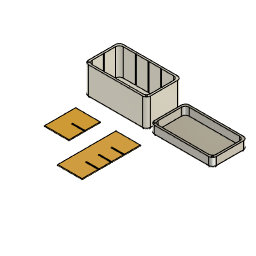
modularTreatBox v3 (Autodesk Fusion 360 design; units mm, degrees)
Autodesk Fusion 360 part; units mm, degrees
note: some values were not read from the file. Chosen so that the rebuilt part matches the saved one: which face or edge a step refers to.
sketch "Sketch1" plane through (0, 0, 0) normal (0, 0, 1) x (1, 0, 0)
  line L0 (65, 40) -> (-65, 40)
  line L1 (-75, 30) -> (-75, -30)
  line L2 (-65, -40) -> (65, -40)
  line L3 (75, -30) -> (75, 30)
  line L4 (-70, 45) -> (70, 45)
  line L5 (80, 35) -> (80, -35)
  line L6 (70, -45) -> (-70, -45)
  line L7 (-80, -35) -> (-80, 35)
  arc A0 (-65, 40) -> (-75, 30) centre (-65, 30) ccw
  arc A1 (-75, -30) -> (-65, -40) centre (-65, -30) ccw
  arc A2 (65, -40) -> (75, -30) centre (65, -30) ccw
  arc A3 (75, 30) -> (65, 40) centre (65, 30) ccw
  arc A4 (70, -45) -> (80, -35) centre (70, -35) ccw
  arc A5 (80, 35) -> (70, 45) centre (70, 35) ccw
  arc A6 (-70, 45) -> (-80, 35) centre (-70, 35) ccw
  arc A7 (-80, -35) -> (-70, -45) centre (-70, -35) ccw
  point P0 (75, 40)
  point P1 (-75, 40)
  point P2 (75, -40)
  point P3 (-80, 45)
  point P4 (80, 45)
  point P5 (-80, -45)
  dimension "d3" = 150
  dimension "d4" = 80
  dimension "d7" = 160
  dimension "d8" = 90
  dimension "d9" = 10
  dimension "d10" = 10
  dimension "d11" = 10
  constraint horizontal L0
  constraint vertical L1
  constraint horizontal L2
  constraint vertical L3
  constraint horizontal L4
  constraint vertical L5
  constraint horizontal L6
  constraint vertical L7
  constraint coincident P1 L0
  constraint coincident P1 L1
  constraint tangent L0 A0
  constraint tangent L1 A0
  constraint tangent L1 A1
  constraint tangent L2 A1
  constraint coincident P2 L2
  constraint coincident P2 L3
  constraint tangent L2 A2
  constraint tangent L3 A2
  constraint equal A1 A2
  constraint coincident P0 L0
  constraint coincident P0 L3
  constraint tangent L0 A3
  constraint tangent L3 A3
  constraint equal A1 A3
  constraint tangent L5 A4
  constraint tangent L6 A4
  constraint coincident P4 L4
  constraint coincident P4 L5
  constraint tangent L4 A5
  constraint tangent L5 A5
  constraint equal A4 A5
  constraint coincident P3 L4
  constraint coincident P3 L7
  constraint tangent L4 A6
  constraint tangent L7 A6
  constraint equal A4 A6
  constraint coincident P5 L6
  constraint coincident P5 L7
  constraint tangent L6 A7
  constraint tangent L7 A7
  constraint equal A4 A7
  measures "d3" distance of P0 P1
  measures "d4" distance of P0 P2
  measures "d7" distance of P3 P4
  measures "d8" distance of P3 P5
  measures "d9" radius of A0
  measures "d10" radius of A1
  measures "d11" radius of A4
extrude "Extrude1" add sketch "Sketch1" against normal blind 5 contours L0 L1 L2 L3 A0 A1 A2 A3 | L4 L5 L6 L7 A4 A5 A6 A7 makes body 1
extrude "Extrude2" add sketch "Sketch1" along normal blind 70 bodies 1
copy_body "CopyPasteBodies1" bodies 1 makes body 2
move_body "Move1" bodies 2 to x (1, 0, 0) y (0, 1, 0) z (0, 0, 1) at (170, 0, 0)
extrude "Extrude3" cut 1 faces at (191.6667, -43.3333, 70) along direction (0, 0, -1) blind 50 on bodies 2 bodies 2
sketch "Sketch2" plane through (0, 0, 70) normal (0, 0, 1) x (-1, 0, 0)
  arc A0 (-75, -30) -> (-65, -40) centre (-65, -30) ccw
  line L0 (-75, -30) -> (-75, 30)
  arc A1 (-65, 40) -> (-75, 30) centre (-65, 30) ccw
  line L1 (-65, 40) -> (65, 40)
  arc A2 (75, 30) -> (65, 40) centre (65, 30) ccw
  line L2 (75, 30) -> (75, -30)
  arc A3 (65, -40) -> (75, -30) centre (65, -30) ccw
  line L3 (65, -40) -> (-65, -40)
  arc A4 (70, -45) -> (80, -35) centre (70, -35) ccw
  line L4 (80, -35) -> (80, 35)
  arc A5 (80, 35) -> (70, 45) centre (70, 35) ccw
  line L5 (70, 45) -> (-70, 45)
  arc A6 (-70, 45) -> (-80, 35) centre (-70, 35) ccw
  line L6 (-80, 35) -> (-80, -35)
  arc A7 (-80, -35) -> (-70, -45) centre (-70, -35) ccw
  line L7 (-70, -45) -> (70, -45)
  line L8 (65, -40) -> (32.5, -40)
  line L9 (32.5, -40) -> (0, -40)
  line L10 (0, -40) -> (-32.5, -40)
  line L11 (-32.5, -40) -> (-65, -40)
  line L12 (32.5, -40) -> (32.5, 40)
  line L13 (0, -40) -> (0, 40)
  line L14 (-32.5, -40) -> (-32.5, 40)
  line L15 (-75, 0) -> (75, 0)
  arc A8 (75, -1.25) -> (75, 1.25) centre (75, 0) ccw
  arc A9 (31.25, -40) -> (33.75, -40) centre (32.5, -40) ccw
  arc A10 (-1.25, -40) -> (1.25, -40) centre (0, -40) ccw
  arc A11 (-33.75, -40) -> (-31.25, -40) centre (-32.5, -40) ccw
  arc A12 (-31.25, 40) -> (-33.75, 40) centre (-32.5, 40) ccw
  arc A13 (1.25, 40) -> (-1.25, 40) centre (0, 40) ccw
  arc A14 (33.75, 40) -> (31.25, 40) centre (32.5, 40) ccw
  arc A15 (-75, 1.25) -> (-75, -1.25) centre (-75, 0) ccw
  dimension "d18" = 32.5
  dimension "d19" = 32.5
  dimension "d20" = 32.5
  dimension "d21" = 1.25
  dimension "d22" = 1.25
  dimension "d23" = 1.25
  dimension "d24" = 1.25
  dimension "d25" = 1.25
  dimension "d26" = 1.25
  dimension "d27" = 1.25
  dimension "d28" = 1.25
  constraint coincident A3.start L3.start
  constraint parallel L3 L8
  constraint parallel L3 L9
  constraint parallel L3 L10
  constraint coincident A0.end L3.end
  constraint coincident L1 L12.end
  constraint perpendicular L1 L12
  constraint midpoint L1 L13.end
  constraint coincident L1 L14.end
  constraint perpendicular L1 L14
  constraint midpoint L0 L15.start
  constraint midpoint L2 L15.end
  constraint coincident L2 A8.end
  constraint coincident L2 A8.start
  constraint coincident L15.end A8.centre
  constraint coincident L8 A9.start
  constraint coincident L8.end L9.start
  constraint coincident L9 A10.start
  constraint coincident L9.end L10.start
  constraint coincident L10 A11.start
  constraint coincident L10.end L11.start
  constraint coincident L1 A12.start
  constraint coincident L14.end A12.centre
  constraint coincident L1 A13.start
  constraint coincident L13.end A13.centre
  constraint coincident L1 A14.start
  constraint coincident L12.end A14.centre
  constraint coincident L0 A15.start
  constraint coincident L15.start A15.centre
  measures "d18" distance of A3.start L8.end
  measures "d19" distance of L8.end L9.end
  measures "d20" distance of L9.end L10.end
  measures "d21" radius of A8
  measures "d22" radius of A9
  measures "d23" radius of A10
  measures "d24" radius of A11
  measures "d25" radius of A12
  measures "d26" radius of A13
  measures "d27" radius of A14
  measures "d28" radius of A15
extrude "Extrude4" cut sketch "Sketch2" against normal blind 70 contours L0 A15 | L3 L10 L11 A11 | L3 L9 L10 A10 | L1 A12 | L1 A13 | L3 L8 L9 A9 | L1 A14 | L2 A8 bodies 1
sketch "Sketch3" plane through (0, 0, 0) normal (0, 0, 1) x (1, 0, 0)
  line L0 (-59.1525, -89.47) -> (5.8475, -89.47)
  line L1 (5.8475, -89.47) -> (5.8475, -169.47)
  line L2 (5.8475, -169.47) -> (-59.1525, -169.47)
  line L3 (-59.1525, -169.47) -> (-59.1525, -89.47)
  line L4 (44.5193, -89.47) -> (109.5193, -89.47)
  line L5 (109.5193, -89.47) -> (109.5193, -239.47)
  line L6 (109.5193, -239.47) -> (44.5193, -239.47)
  line L7 (44.5193, -239.47) -> (44.5193, -89.47)
  line L8 (5.8475, -129.47) -> (-26.6525, -129.47)
  line L9 (-75, -30, 70) -> (-75, -1.25, 70)
  line L10 (-33.75, -40, 70) -> (-65, -40, 70)
  line L11 (-75, -1.25, 70) -> (-75, -62.1783, 70)
  line L12 (-33.75, -40, 70) -> (-75, -40, 70)
  dimension "d31" = 65
  dimension "d32" = 80
  dimension "d33" = 65
  dimension "d34" = 150
  dimension "d35" = 32.5
  constraint horizontal L0
  constraint vertical L1
  constraint horizontal L2
  constraint vertical L3
  constraint horizontal L4
  constraint vertical L5
  constraint horizontal L6
  constraint vertical L7
  constraint midpoint L1 L8.start
  constraint perpendicular L3 L8
  measures "d31" distance of L0.start L0.end
  measures "d32" distance of L0.start L2.end
  measures "d33" distance of L4.start L4.end
  measures "d34" distance of L4.start L6.end
  measures "d35" distance of L8.start L8.end
sketch "Sketch4" plane through (0, 0, 0) normal (0, 0, 1) x (1, 0, 0)
  line L0 (109.5193, -89.47) -> (109.5193, -131.97)
  line L1 (109.5193, -239.47) -> (109.5193, -196.97)
  line L2 (109.5193, -89.47) -> (109.5193, -239.47)
  line L3 (109.5193, -164.47) -> (77.0193, -164.47)
  line L4 (109.5193, -131.97) -> (77.0193, -131.97)
  line L5 (109.5193, -196.97) -> (77.0193, -196.97)
  line L6 (109.5193, -195.72) -> (77.0193, -195.72)
  line L7 (77.0193, -195.72) -> (77.0193, -198.22)
  line L8 (77.0193, -198.22) -> (109.5193, -198.22)
  line L9 (109.5193, -198.22) -> (109.5193, -195.72)
  line L10 (109.5193, -195.72) -> (77.0193, -198.22) construction
  line L11 (77.0193, -195.72) -> (109.5193, -198.22) construction
  line L12 (109.5193, -163.22) -> (77.0193, -163.22)
  line L13 (77.0193, -163.22) -> (77.0193, -165.72)
  line L14 (77.0193, -165.72) -> (109.5193, -165.72)
  line L15 (109.5193, -165.72) -> (109.5193, -163.22)
  line L16 (109.5193, -163.22) -> (77.0193, -165.72) construction
  line L17 (77.0193, -163.22) -> (109.5193, -165.72) construction
  line L18 (109.5193, -130.72) -> (77.0193, -130.72)
  line L19 (77.0193, -130.72) -> (77.0193, -133.22)
  line L20 (77.0193, -133.22) -> (109.5193, -133.22)
  line L21 (109.5193, -133.22) -> (109.5193, -130.72)
  line L22 (109.5193, -130.72) -> (77.0193, -133.22) construction
  line L23 (77.0193, -130.72) -> (109.5193, -133.22) construction
  line L24 (5.8475, -128.22) -> (-26.6525, -128.22)
  line L25 (-26.6525, -128.22) -> (-26.6525, -130.72)
  line L26 (-26.6525, -130.72) -> (5.8475, -130.72)
  line L27 (5.8475, -130.72) -> (5.8475, -128.22)
  line L28 (5.8475, -128.22) -> (-26.6525, -130.72) construction
  line L29 (-26.6525, -128.22) -> (5.8475, -130.72) construction
  line L30 (5.8475, -129.47) -> (-26.6525, -129.47)
  arc A0 (-26.6525, -128.22) -> (-26.6525, -130.72) centre (-26.6525, -129.47) ccw
  arc A1 (77.0193, -130.72) -> (77.0193, -133.22) centre (77.0193, -131.97) ccw
  arc A2 (77.0193, -163.22) -> (77.0193, -165.72) centre (77.0193, -164.47) ccw
  arc A3 (77.0193, -195.72) -> (77.0193, -198.22) centre (77.0193, -196.97) ccw
  line L31 (5.8475, -128.22) -> (5.8475, -130.72)
  line L32 (109.5193, -130.72) -> (109.5193, -198.22)
  point P0 (109.5193, -89.47)
  point P1 (109.5193, -239.47)
  point P2 (93.2693, -196.97)
  point P3 (93.2693, -164.47)
  point P4 (93.2693, -131.97)
  point P5 (-10.4025, -129.47)
  constraint coincident P0 L0.start
  constraint coincident P1 L1.start
  constraint midpoint L2 L3.start
  constraint perpendicular L0 L3
  constraint perpendicular L2 L4
  constraint perpendicular L1 L5
  constraint horizontal L6
  constraint perpendicular L6 L7
  constraint parallel L6 L8
  constraint parallel L7 L9
  constraint coincident L10 P2
  constraint coincident L11 P2
  constraint coincident L2 L6.start
  constraint midpoint L5 P2
  constraint horizontal L12
  constraint perpendicular L12 L13
  constraint parallel L12 L14
  constraint parallel L13 L15
  constraint coincident L16 P3
  constraint coincident L17 P3
  constraint coincident L2 L12.start
  constraint midpoint L3 P3
  constraint horizontal L18
  constraint perpendicular L18 L19
  constraint parallel L18 L20
  constraint parallel L19 L21
  constraint coincident L22 P4
  constraint coincident L23 P4
  constraint midpoint L4 P4
  constraint horizontal L24
  constraint perpendicular L24 L25
  constraint parallel L24 L26
  constraint parallel L25 L27
  constraint coincident L28 P5
  constraint coincident L29 P5
  constraint midpoint P5 L30
  constraint coincident L30.end A0.centre
  constraint coincident L4.end A1.centre
  constraint coincident L3.end A2.centre
  constraint coincident L5.end A3.centre
  constraint perpendicular L8 L32
extrude "Extrude5" add sketch "Sketch3" along normal blind 2 separate body makes body 3 at (-15.8192, -142.8033, 0) makes body 4 at (66.186, -139.47, 0)
extrude "Extrude6" cut sketch "Sketch4" along normal blind 10 bodies 3 4
sketch "Sketch5" plane through (44.5193, 0, 0) normal (-1, 0, 0) x (0, -1, 0)
  line L0 (89.47, 0) -> (239.47, 0)
  line L1 (239.47, 0) -> (239.47, 2)
  line L2 (239.47, 2) -> (89.47, 2)
  line L3 (89.47, 2) -> (89.47, 0)
  arc A0 (239.47, 0) -> (239.47, 2) centre (239.47, 1) ccw
  arc A1 (89.47, 2) -> (89.47, 0) centre (89.47, 1) ccw
  arc A2 through (89.47, 2, 103.6719) (88.47, 1, 103.6719) (89.47, 0, 103.6719)
  line L4 (89.47, 0, 103.6719) -> (89.47, 2, 103.6719)
  arc A3 through (169.47, 0, 103.6719) (170.47, 1, 103.6719) (169.47, 2, 103.6719)
  line L5 (169.47, 0, 103.6719) -> (169.47, 2, 103.6719)
  point P0 (89.47, 2)
  point P1 (89.47, 0)
  point P2 (169.47, 0)
  point P3 (169.47, 2)
  constraint coincident L0.end L1.start
  constraint coincident L1.end L2.start
  constraint midpoint L1 A0.centre
  constraint coincident L0.start L3.end
  constraint coincident P0 L2.end
  constraint midpoint L3 A1.centre
  constraint coincident P1 L0.start
sketch "Sketch5 (curves 103.6719 mm off its plane)" plane through (-59.1526, 0, 0) normal (-1, 0, 0) x (0, -1, 0)
  arc A0 (89.47, 2) -> (89.47, 0) centre (89.47, 1) ccw
  line L0 (89.47, 0) -> (89.47, 2)
  arc A1 (169.47, 0) -> (169.47, 2) centre (169.47, 1) ccw
  line L1 (169.47, 0) -> (169.47, 2)
extrude "Extrude7" add sketch "Sketch5 (curves 103.6719 mm off its plane)" against normal blind 65 bodies 3
extrude "Extrude8" add sketch "Sketch5" against normal blind 65 contours L3 A1 | L1 A0 bodies 4
fillet "Fillet1" radius 1 4 edges at (44.5193, -240.47, 1) (44.5193, -164.47, 0) (44.5193, -88.47, 1) (44.5193, -164.47, 2) on bodies 4
fillet "Fillet2" radius 1 24 edges at (-59.1525, -129.47, 0) (-59.1525, -129.47, 2) (-59.1526, -170.47, 1) (-59.1526, -88.47, 1) (5.8475, -108.845, 0) (5.8475, -150.095, 0) (5.8475, -108.845, 2) (5.8475, -150.095, 2) (5.8474, -170.47, 1) (5.8474, -88.47, 1) (109.5193, -110.095, 2) (109.5193, -218.845, 2) (109.5193, -148.22, 2) (109.5193, -180.72, 2) (109.5193, -110.095, 0) (109.5193, -218.845, 0) (109.5193, -148.22, 0) (109.5193, -180.72, 0) (109.5193, -240.47, 1) (109.5193, -88.47, 1) (109.5193, -133.22, 1) (109.5193, -163.22, 1) (109.5193, -195.72, 1) (109.5193, -165.72, 1) on bodies 3 4
sketch "Sketch6" plane through (0, 0, 70) normal (0, 0, 1) x (-1, 0, 0)
  arc A0 (70, -45) -> (80, -35) centre (70, -35) ccw
  line L0 (80, -35) -> (80, 35)
  arc A1 (80, 35) -> (70, 45) centre (70, 35) ccw
  line L1 (70, 45) -> (-70, 45)
  arc A2 (-70, 45) -> (-80, 35) centre (-70, 35) ccw
  line L2 (-80, 35) -> (-80, -35)
  arc A3 (-80, -35) -> (-70, -45) centre (-70, -35) ccw
  line L3 (-70, -45) -> (70, -45)
  arc A4 (1.25, 40) -> (-1.25, 40) centre (0, 40) ccw
  line L4 (1.25, 40) -> (31.25, 40)
  arc A5 (33.75, 40) -> (31.25, 40) centre (32.5, 40) ccw
  line L5 (33.75, 40) -> (65, 40)
  arc A6 (75, 30) -> (65, 40) centre (65, 30) ccw
  line L6 (75, 30) -> (75, 1.25)
  arc A7 (75, -1.25) -> (75, 1.25) centre (75, 0) ccw
  line L7 (75, -1.25) -> (75, -30)
  arc A8 (65, -40) -> (75, -30) centre (65, -30) ccw
  line L8 (65, -40) -> (33.75, -40)
  arc A9 (31.25, -40) -> (33.75, -40) centre (32.5, -40) ccw
  line L9 (31.25, -40) -> (1.25, -40)
  arc A10 (-1.25, -40) -> (1.25, -40) centre (0, -40) ccw
  line L10 (-1.25, -40) -> (-31.25, -40)
  arc A11 (-33.75, -40) -> (-31.25, -40) centre (-32.5, -40) ccw
  line L11 (-33.75, -40) -> (-65, -40)
  arc A12 (-75, -30) -> (-65, -40) centre (-65, -30) ccw
  line L12 (-75, -30) -> (-75, -1.25)
  arc A13 (-75, 1.25) -> (-75, -1.25) centre (-75, 0) ccw
  line L13 (-75, 1.25) -> (-75, 30)
  arc A14 (-65, 40) -> (-75, 30) centre (-65, 30) ccw
  line L14 (-65, 40) -> (-33.75, 40)
  arc A15 (-31.25, 40) -> (-33.75, 40) centre (-32.5, 40) ccw
  line L15 (-31.25, 40) -> (-1.25, 40)
  circle A16 centre (-74.5711, 39.5711) radius 2.025
  circle A17 centre (74.7989, 39.3275) radius 2.025
  dimension "d57" = 4.05
  dimension "d58" = 4.05
  measures "d57" diameter of A16
  measures "d58" diameter of A17
sketch "Sketch7" plane through (0, 0, 20) normal (0, 0, 1) x (-1, 0, 0)
  arc A0 (-245, -30) -> (-235, -40) centre (-235, -30) ccw
  line L0 (-245, -30) -> (-245, 30)
  arc A1 (-235, 40) -> (-245, 30) centre (-235, 30) ccw
  line L1 (-235, 40) -> (-105, 40)
  arc A2 (-95, 30) -> (-105, 40) centre (-105, 30) ccw
  line L2 (-95, 30) -> (-95, -30)
  arc A3 (-105, -40) -> (-95, -30) centre (-105, -30) ccw
  line L3 (-105, -40) -> (-235, -40)
  arc A4 (-100, -45) -> (-90, -35) centre (-100, -35) ccw
  line L4 (-90, -35) -> (-90, 35)
  arc A5 (-90, 35) -> (-100, 45) centre (-100, 35) ccw
  line L5 (-100, 45) -> (-240, 45)
  arc A6 (-240, 45) -> (-250, 35) centre (-240, 35) ccw
  line L6 (-250, 35) -> (-250, -35)
  arc A7 (-250, -35) -> (-240, -45) centre (-240, -35) ccw
  line L7 (-240, -45) -> (-100, -45)
  circle A8 centre (-95.4289, 39.5711) radius 2.025
  circle A9 centre (-244.5711, 39.5711) radius 2.025
  dimension "d59" = 4.05
  dimension "d60" = 4.05
  measures "d59" diameter of A8
  measures "d60" diameter of A9
extrude "Extrude9" cut sketch "Sketch6" against normal blind 10 contours A16 | A17 bodies 1
extrude "Extrude10" cut sketch "Sketch7" against normal blind 10 contours A8 | A9 bodies 2
fillet "Fillet3" radius 5 2 faces at (23.3333, -15, -5) (193.3333, -15, -5) on bodies 1 2
equation "d18 = ( 130 / 4 ) * 1 mm"
named bodies: "Body", "Lid", "Short", "Long"
